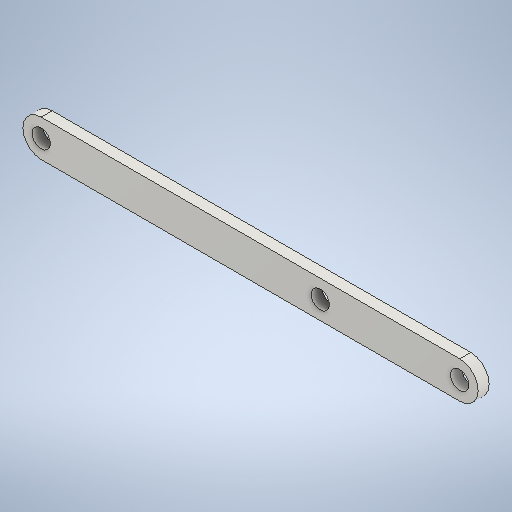
# Autodesk Inventor part: 31 - Lever
Saved by Autodesk Inventor 2025.2 (Build 292293000, 293)
## iProperties
Created: 2025-07-17
Part Number: 31 - Lever
Material: Steel AISI 1020 108 ANLD
Document SubType Name: Modeling
Designer: bless
Density: 7.87 g/cm^3
Appearance: Steel
Author: bless
Autodesk Inventor part; units mm, degrees
ref_plane "YZ Plane" through (0, 0, 0) normal (1, 0, 0) x (0, 1, 0)
ref_plane "XZ Plane" through (0, 0, 0) normal (0, 1, 0) x (-1, 0, 0)
ref_plane "XY Plane" through (0, 0, 0) normal (0, 0, 1) x (1, 0, 0)
sketch "Sketch1" plane through (0, 0, 0) normal (0, 0, 1) x (1, 0, 0)
  arc A0 (0, -2.5) -> (0, 2.5) centre (0, 0) ccw
  arc A1 (-57, 2.5) -> (-57, -2.5) centre (-57, 0) ccw
  line L0 (-57, 2.5) -> (0, 2.5)
  line L1 (0, -2.5) -> (-57, -2.5)
  dimension "d0" = 2.5
  dimension "d1" = 2.5
  dimension "d2" = 57
  constraints: 4 end point, 4 point on circle, 4 tangent, 2 centre point, 1 coincident, 1 horizontal alignment
  measures "d0" radius of A0
  measures "d1" radius of A1
  measures "d2" distance of point (0, 0) A1.centre
extrude "Extrusion1" add sketch "Sketch1" along normal blind 1.5
sketch "Sketch2" plane through (0, 0, 1.5) normal (0, 0, 1) x (1, 0, 0)
  arc A0 (0, -2.5) -> (0, 2.5) centre (0, 0) ccw projected
  arc A1 (-57, 2.5) -> (-57, -2.5) centre (-57, 0) ccw projected
  point P0 (-19, 0)
  dimension "d5" = 38
  dimension "d6" = 19
  constraints: 2 coincident
  measures "d5" distance of A1.centre point (-19, 0)
  measures "d6" distance of point (-19, 0) A0.centre
hole "Hole1" at (-57, 0, 1.5) at (-19, 0, 1.5) at (0, 0, 1.5) direction (0, 0, -1) diameter 2.5 end through all
body "Solid1"
